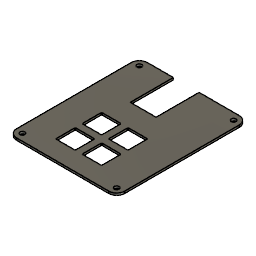
HeackYeahdee (Autodesk Fusion 360 design; units mm, degrees)
part number: 2025-12-04-21-24-05-304
Autodesk Fusion 360 part; units mm, degrees
sketch "plate-2025-12-04T13_16_58.583Z" plane through (0, 0, 0) normal (0, 0, 1) x (1, 0, 0)
  line L0 (3.025, -21.575) -> (16.025, -21.575)
  line L1 (3.025, -35.575) -> (16.025, -35.575)
  line L2 (2.525, -22.075) -> (2.525, -35.075)
  line L3 (16.525, -22.075) -> (16.525, -35.075)
  arc A0 (3.025, -21.575) -> (2.525, -22.075) centre (3.025, -22.075) ccw
  arc A1 (16.525, -22.075) -> (16.025, -21.575) centre (16.025, -22.075) ccw
  arc A2 (2.525, -35.075) -> (3.025, -35.575) centre (3.025, -35.075) ccw
  arc A3 (16.025, -35.575) -> (16.525, -35.075) centre (16.025, -35.075) ccw
  line L4 (22.075, -21.575) -> (35.075, -21.575)
  line L5 (22.075, -35.575) -> (35.075, -35.575)
  line L6 (21.575, -22.075) -> (21.575, -35.075)
  line L7 (35.575, -22.075) -> (35.575, -35.075)
  arc A4 (22.075, -21.575) -> (21.575, -22.075) centre (22.075, -22.075) ccw
  arc A5 (35.575, -22.075) -> (35.075, -21.575) centre (35.075, -22.075) ccw
  arc A6 (21.575, -35.075) -> (22.075, -35.575) centre (22.075, -35.075) ccw
  arc A7 (35.075, -35.575) -> (35.575, -35.075) centre (35.075, -35.075) ccw
  line L8 (3.025, -40.625) -> (16.025, -40.625)
  line L9 (3.025, -54.625) -> (16.025, -54.625)
  line L10 (2.525, -41.125) -> (2.525, -54.125)
  line L11 (16.525, -41.125) -> (16.525, -54.125)
  arc A8 (3.025, -40.625) -> (2.525, -41.125) centre (3.025, -41.125) ccw
  arc A9 (16.525, -41.125) -> (16.025, -40.625) centre (16.025, -41.125) ccw
  arc A10 (2.525, -54.125) -> (3.025, -54.625) centre (3.025, -54.125) ccw
  arc A11 (16.025, -54.625) -> (16.525, -54.125) centre (16.025, -54.125) ccw
  line L12 (22.075, -40.625) -> (35.075, -40.625)
  line L13 (22.075, -54.625) -> (35.075, -54.625)
  line L14 (21.575, -41.125) -> (21.575, -54.125)
  line L15 (35.575, -41.125) -> (35.575, -54.125)
  arc A12 (22.075, -40.625) -> (21.575, -41.125) centre (22.075, -41.125) ccw
  arc A13 (35.575, -41.125) -> (35.075, -40.625) centre (35.075, -41.125) ccw
  arc A14 (21.575, -54.125) -> (22.075, -54.625) centre (22.075, -54.125) ccw
  arc A15 (35.075, -54.625) -> (35.575, -54.125) centre (35.075, -54.125) ccw
  line L16 (0, -57.15) -> (38.1, -57.15)
  line L17 (0, -19.05) -> (38.1, -19.05)
  line L18 (0, -57.15) -> (0, -19.05)
  line L19 (38.1, -57.15) -> (38.1, -19.05)
  line L20 (-17.994, 26.134) -> (60.006, 26.134)
  line L21 (60.006, 26.134) -> (60.006, -68.197)
  line L22 (60.006, -68.197) -> (-17.994, -68.197)
  line L23 (-17.994, -68.197) -> (-17.994, 26.134)
  line L24 (6.604, 26.134) -> (25.104, 26.134)
  line L25 (25.104, 26.134) -> (25.104, -4.866)
  line L26 (25.104, -4.866) -> (6.604, -4.866)
  line L27 (6.604, -4.866) -> (6.604, 26.134)
  circle A16 centre (-12.994, 21.134) radius 1.7
  circle A17 centre (55.006, 21.134) radius 1.7
  circle A18 centre (-12.994, -63.197) radius 1.7
  circle A19 centre (55.006, -63.197) radius 1.7
  dimension "d1" = 78
  dimension "d2" = 94.331
  dimension "d4" = 20.519
  dimension "d5" = 13.572
  dimension "d6" = 18.5
  dimension "d7" = 31
  dimension "d8" = 24.598
  dimension "d9" = 3.4
  dimension "d10" = 5
  dimension "d11" = 5
  dimension "d12" = 3.4
  dimension "d13" = 5
  dimension "d14" = 5
  dimension "d15" = 3.4
  dimension "d16" = 5
  dimension "d17" = 5
  dimension "d18" = 3.4
  dimension "d19" = 5
  dimension "d20" = 5
  constraint horizontal L20
  constraint vertical L21
  constraint horizontal L22
  constraint vertical L23
  constraint horizontal L24
  constraint vertical L25
  constraint horizontal L26
  constraint vertical L27
  constraint coincident L20 L24.start
  measures "d1" distance of L21 L23
  measures "d2" distance of L20 L22
  measures "d4" distance of L10 L23
  measures "d5" distance of L9 L22
  measures "d6" distance of L25 L27
  measures "d7" distance of L24 L26
  measures "d8" distance of L23 L27
  measures "d9" diameter of A16
  measures "d10" distance of L20 A16.centre
  measures "d11" distance of L23 A16.centre
  measures "d12" diameter of A17
  measures "d13" distance of L20 A17.centre
  measures "d14" distance of L21 A17.centre
  measures "d15" diameter of A18
  measures "d16" distance of L22 A18.centre
  measures "d17" distance of L23 A18.centre
  measures "d18" diameter of A19
  measures "d19" distance of L22 A19.centre
  measures "d20" distance of L21 A19.centre
extrude "Extrude1" add sketch "plate-2025-12-04T13_16_58.583Z" along normal blind 1.5 contours L16 L17 L18 L19 | L20 L21 L22 L23 L25 L26 L27
fillet "Fillet1" radius 5.75 1 edges at (60.006, -68.197, 0.75)
fillet "Fillet2" radius 5.75 1 edges at (-17.994, -68.197, 0.75)
fillet "Fillet3" radius 5.75 1 edges at (60.006, 26.134, 0.75)
fillet "Fillet4" radius 5.75 1 edges at (-17.994, 26.134, 0.75)
equation "d5 = 9.5 mm + 4.072 mm"
equation "d8 = 18.848 mm + 5.75 mm"
